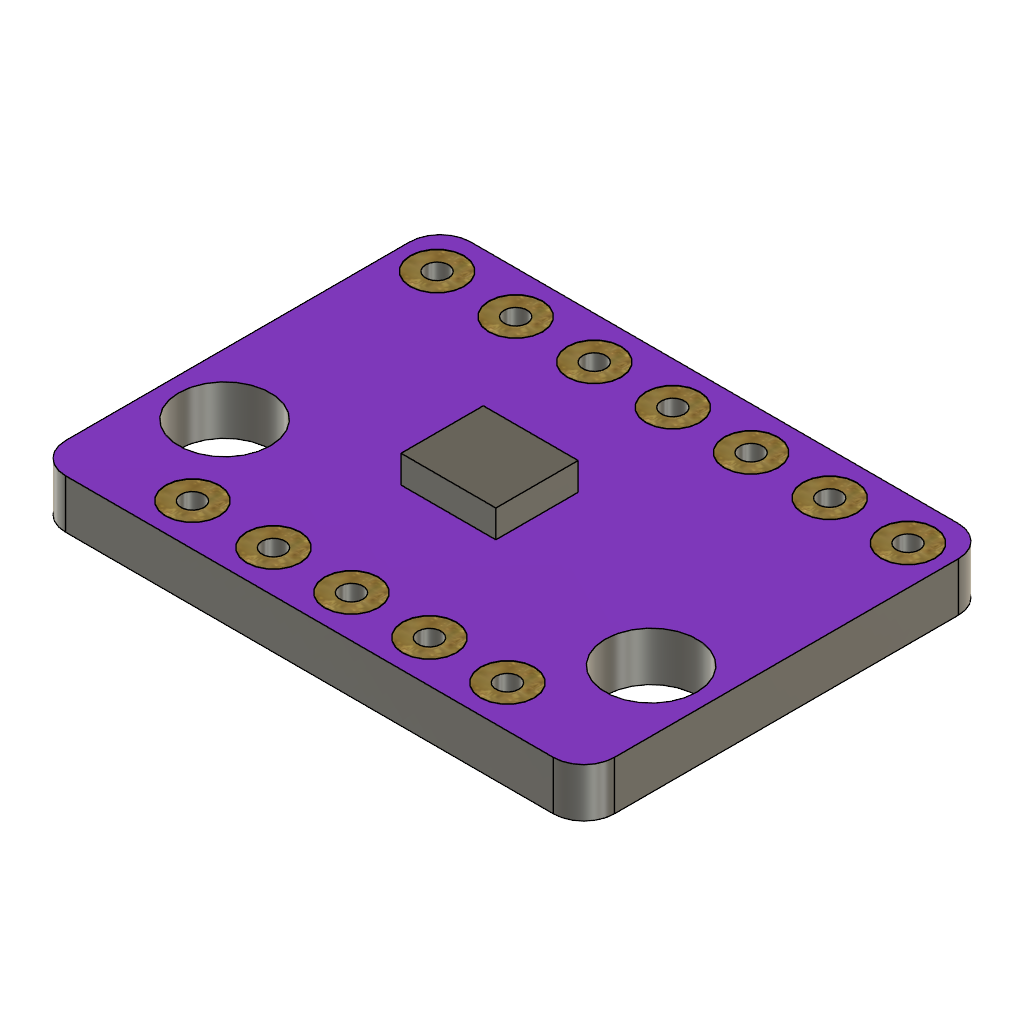
bmi160 (Autodesk Fusion 360 design; units mm, degrees)
Autodesk Fusion 360 part; units mm, degrees
sketch "Sketch2" plane through (0, 0, 0) normal (0, 0, 1) x (1, 0, 0)
  line L0 (-8.9478, 7.7363) -> (9.0022, 7.7363)
  line L1 (9.0022, 7.7363) -> (9.0022, -5.5137)
  line L2 (9.0022, -5.5137) -> (-8.9478, -5.5137)
  line L3 (-8.9478, -5.5137) -> (-8.9478, 7.7363)
  line L4 (-8.9478, 7.7363) -> (9.0022, -5.5137) construction
  line L5 (-8.9478, -5.5137) -> (9.0022, 7.7363) construction
  line L6 (-9.5685, 6.7363) -> (10, 6.7363) construction
  line L7 (-9.5685, 6.3613) -> (10, 6.3613) construction
  line L8 (-10.5, -4.5137) -> (10.5, -4.5137) construction
  line L9 (-10.5, -4.1387) -> (10.5, -4.1387) construction
  line L10 (8.5022, 9) -> (8.5022, -6.5) construction
  line L11 (7.0022, 9) -> (7.0022, -6.5) construction
  line L12 (-8.4478, 9.5) -> (-8.4478, -7) construction
  line L13 (-6.9478, 9.5) -> (-6.9478, -7) construction
  line L14 (-10.5, -2.8137) -> (11.6299, -2.8137) construction
  line L15 (-10.5, -1.3137) -> (11.6299, -1.3137) construction
  circle A0 centre (7.0022, -1.3137) radius 1.5
  circle A1 centre (-6.9478, -1.3137) radius 1.5
  line L16 (-8.0478, 9) -> (-8.0478, 5) construction
  line L17 (-7.6728, 9) -> (-7.6728, 5) construction
  circle A2 centre (-7.6728, 6.3613) radius 0.375
  line L18 (-5.1028, 7.3) -> (-5.1028, 4.898) construction
  circle A3 centre (-5.1028, 6.3613) radius 0.375
  circle A4 centre (-2.5328, 6.3613) radius 0.375
  circle A5 centre (0.0372, 6.3613) radius 0.375
  circle A6 centre (2.5972, 6.3613) radius 0.375
  circle A7 centre (5.1672, 6.3613) radius 0.375
  circle A8 centre (7.7272, 6.3613) radius 0.375
  circle A9 centre (-7.6728, 6.3613) radius 0.875
  line L19 (-5.5478, -3.163) -> (-5.5478, -6) construction
  line L20 (-5.1728, -3.163) -> (-5.1728, -6) construction
  circle A10 centre (-5.1728, -4.1387) radius 0.375
  line L21 (-2.1478, -3.7) -> (-2.1478, -5.9) construction
  circle A11 centre (-2.5228, -4.1387) radius 0.375
  line L22 (-2.8978, -3.7) -> (-2.8978, -5.1) construction
  line L23 (0.4022, -3.6) -> (0.4022, -5.1) construction
  circle A12 centre (0.0272, -4.1387) radius 0.375
  line L24 (-0.3478, -3.6) -> (-0.3478, -5.3) construction
  circle A13 centre (2.5772, -4.1387) radius 0.375
  circle A14 centre (5.1272, -4.1387) radius 0.375
  line L25 (2.2022, -3.6) -> (2.2022, -5.1) construction
  line L26 (4.7522, -3.7) -> (4.7522, -5.1) construction
  line L27 (2.9522, -3.8) -> (2.9522, -4.9) construction
  line L28 (5.5022, -3.7) -> (5.5022, -5.1) construction
  circle A15 centre (-5.1028, 6.3613) radius 0.875
  circle A16 centre (-2.5328, 6.3613) radius 0.875
  circle A17 centre (0.0372, 6.3613) radius 0.875
  circle A18 centre (2.5972, 6.3613) radius 0.875
  circle A19 centre (5.1672, 6.3613) radius 0.875
  circle A20 centre (7.7272, 6.3613) radius 0.875
  circle A21 centre (5.1272, -4.1387) radius 0.875
  circle A22 centre (2.5772, -4.1387) radius 0.875
  circle A23 centre (0.0272, -4.1387) radius 0.875
  circle A24 centre (-2.5228, -4.1387) radius 0.875
  circle A25 centre (-5.1728, -4.1387) radius 0.875
  line L29 (-2.2, 2.4) -> (0.9, 2.4)
  line L30 (0.9, 2.4) -> (0.9, -0.2901)
  line L31 (0.9, -0.2901) -> (-2.2, -0.2901)
  line L32 (-2.2, -0.2901) -> (-2.2, 2.4)
  dimension "d1" = 17.95
  dimension "d2" = 13.25
  dimension "d3" = 1
  dimension "d4" = 0.375
  dimension "d5" = 1
  dimension "d6" = -0.375
  dimension "d7" = 0.5
  dimension "d8" = 1.5
  dimension "d9" = 0.5
  dimension "d10" = -1.5
  dimension "d11" = 2.7
  dimension "d12" = -1.5
  dimension "d13" = 3
  dimension "d14" = 3
  dimension "d15" = 0.9
  dimension "d17" = 0.75
  dimension "d19" = 2.57
  dimension "d21" = 0.75
  dimension "d22" = 0.75
  dimension "d23" = 2.57
  dimension "d24" = 0.75
  dimension "d25" = 2.57
  dimension "d26" = 0.75
  dimension "d27" = 2.56
  dimension "d28" = 0.75
  dimension "d29" = 2.57
  dimension "d30" = 0.75
  dimension "d31" = 2.56
  dimension "d32" = 0.5
  dimension "d33" = 3.4
  dimension "d34" = -0.375
  dimension "d35" = 0.75
  dimension "d36" = 3.4
  dimension "d37" = 0.75
  dimension "d38" = 0.75
  dimension "d39" = 3.3
  dimension "d40" = 0.75
  dimension "d41" = 0.75
  dimension "d42" = 3.3
  dimension "d43" = 3.3
  dimension "d44" = 0.5
  dimension "d45" = 0.5
  dimension "d46" = 0.5
  dimension "d47" = 0.5
  dimension "d48" = 0.5
  dimension "d49" = 0.5
  dimension "d50" = 0.5
  dimension "d51" = 0.5
  dimension "d52" = 0.5
  dimension "d53" = 0.5
  dimension "d54" = 0.5
  constraint horizontal L0
  constraint vertical L1
  constraint horizontal L2
  constraint vertical L3
  constraint perpendicular L1 L6
  constraint perpendicular L3 L8
  constraint perpendicular L2 L10
  constraint perpendicular L2 L12
  constraint perpendicular L10 L14
  constraint coincident L15 A0.centre
  constraint coincident L11 A0.centre
  constraint coincident L15 A1.centre
  constraint coincident L13 A1.centre
  constraint perpendicular L7 L16
  constraint coincident L17 A2.centre
  constraint coincident L7 A2.centre
  constraint coincident L4 L18.end
  constraint perpendicular L6 L18
  constraint coincident L7 A3.centre
  constraint coincident L18 A3.centre
  constraint coincident L7 A4.centre
  constraint coincident L7 A5.centre
  constraint coincident L7 A6.centre
  constraint coincident L7 A7.centre
  constraint coincident L7 A8.centre
  constraint perpendicular L2 L19
  constraint coincident L20 A10.centre
  constraint coincident L9 A10.centre
  constraint perpendicular L2 L21
  constraint coincident L9 A11.centre
  constraint tangent L21 A11
  constraint vertical L22
  constraint tangent A11 L22
  constraint perpendicular L9 L23
  constraint coincident L9 A12.centre
  constraint tangent L23 A12
  constraint perpendicular L8 L24
  constraint tangent A12 L24
  constraint coincident L9 A13.centre
  constraint coincident L9 A14.centre
  constraint vertical L25
  constraint perpendicular L9 L26
  constraint perpendicular L9 L27
  constraint perpendicular L8 L28
  constraint tangent A14 L26
  constraint tangent A14 L28
  constraint tangent A13 L27
  constraint tangent A13 L25
  constraint horizontal L29
  constraint vertical L30
  constraint horizontal L31
  constraint vertical L32
  measures "d1" distance of L0.start L0.end
  measures "d2" distance of L0.start L2.end
  measures "d3" distance of L0 L6
  measures "d5" distance of L2 L8
  measures "d7" distance of L1 L10
  measures "d9" distance of L3 L12
  measures "d11" distance of L2 L14
  measures "d13" diameter of A0
  measures "d14" diameter of A1
  measures "d15" distance of L3 L16
  measures "d17" diameter of A2
  measures "d19" distance of A2.centre L18
  measures "d21" diameter of A3
  measures "d22" diameter of A4
  measures "d23" distance of L18 A4.centre
  measures "d24" diameter of A5
  measures "d25" distance of A4.centre A5.centre
  measures "d26" diameter of A6
  measures "d27" distance of A5.centre A6.centre
  measures "d28" diameter of A7
  measures "d29" distance of A6.centre A7.centre
  measures "d30" diameter of A8
  measures "d31" distance of A7.centre A8.centre
  measures "d33" distance of L3 L19
  measures "d35" diameter of A10
  measures "d36" distance of L19 L21
  measures "d37" diameter of A11
  measures "d38" diameter of A12
  measures "d39" distance of L22 L23
  measures "d40" diameter of A13
  measures "d41" diameter of A14
  measures "d42" distance of L24 L27
  measures "d43" distance of L25 L28
extrude "Extrude1" add sketch "Sketch2" along normal blind 1.6 contours L0 L1 L2 L3 | A9 | A15 | A16 | A17 | A18 | A19 | A20 | A21 | A22 | A23 | A24 | A25 | L29 L30 L31 L32
extrude "Extrude2" add sketch "Sketch2" along normal blind 2.5 contours L29 L30 L31 L32
fillet "Fillet1" radius 1 4 edges at (-8.9478, -5.5137, 0.8) (9.0022, -5.5137, 0.8) (9.0022, 7.7363, 0.8) (-8.9478, 7.7363, 0.8)
sketch "Sketch3" plane through (0, 0, 1.6) normal (0, 0, 1) x (-1, 0, 0)
  line L0 (2.2, 0.2901) -> (2.2, -2.4)
  line L1 (2.2, -2.4) -> (-0.9, -2.4)
  line L2 (-0.9, -2.4) -> (-0.9, 0.2901)
  line L3 (-0.9, 0.2901) -> (2.2, 0.2901)
  circle A0 centre (-2.5972, -6.3613) radius 0.375
  circle A1 centre (-5.1272, 4.1387) radius 0.375
  circle A2 centre (-7.7272, -6.3613) radius 0.375
  circle A3 centre (5.1728, 4.1387) radius 0.375
  circle A4 centre (2.5228, 4.1387) radius 0.375
  circle A5 centre (-5.1672, -6.3613) radius 0.375
  circle A6 centre (-0.0272, 4.1387) radius 0.375
  circle A7 centre (-2.5772, 4.1387) radius 0.375
  circle A8 centre (-0.0372, -6.3613) radius 0.375
  circle A9 centre (2.5328, -6.3613) radius 0.375
  circle A10 centre (7.6728, -6.3613) radius 0.375
  circle A11 centre (6.9478, 1.3137) radius 1.5
  circle A12 centre (5.1028, -6.3613) radius 0.375
  circle A13 centre (-7.0022, 1.3137) radius 1.5
  arc A14 (7.9478, -7.7363) -> (8.9478, -6.7363) centre (7.9478, -6.7363) ccw
  line L4 (8.9478, -6.7363) -> (8.9478, 4.5137)
  arc A15 (8.9478, 4.5137) -> (7.9478, 5.5137) centre (7.9478, 4.5137) ccw
  line L5 (7.9478, 5.5137) -> (-8.0022, 5.5137)
  arc A16 (-8.0022, 5.5137) -> (-9.0022, 4.5137) centre (-8.0022, 4.5137) ccw
  line L6 (-9.0022, 4.5137) -> (-9.0022, -6.7363)
  arc A17 (-9.0022, -6.7363) -> (-8.0022, -7.7363) centre (-8.0022, -6.7363) ccw
  line L7 (-8.0022, -7.7363) -> (7.9478, -7.7363)
  circle A18 centre (-7.7272, -6.3613) radius 0.875
  circle A19 centre (-5.1672, -6.3613) radius 0.875
  circle A20 centre (-2.5972, -6.3613) radius 0.875
  circle A21 centre (-0.0372, -6.3613) radius 0.875
  circle A22 centre (2.5328, -6.3613) radius 0.875
  circle A23 centre (5.1028, -6.3613) radius 0.875
  circle A24 centre (7.6728, -6.3613) radius 0.875
  circle A25 centre (5.1728, 4.1387) radius 0.875
  circle A26 centre (2.5228, 4.1387) radius 0.875
  circle A27 centre (-0.0272, 4.1387) radius 0.875
  circle A28 centre (-2.5772, 4.1387) radius 0.875
  circle A29 centre (-5.1272, 4.1387) radius 0.875
extrude "Extrude3" cut sketch "Sketch3" against normal blind 0.01 contours A18 | A19 | A20 | A21 | A22 | A23 | A24 | A25 | A26 | A27 | A28 | A29
